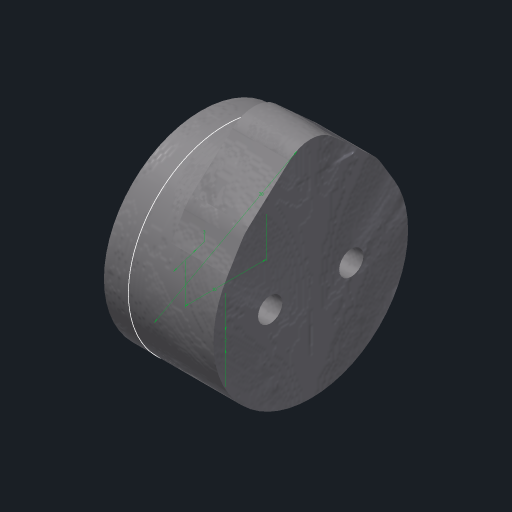
# Autodesk Inventor part: CIRCULAR_FIN_DE_CARRERA
Saved by Autodesk Inventor 2024.3 (Build 283343000, 343)
## iProperties
Created: 2024-07-21
Part Number: CIRCULAR_FIN_DE_CARRERA
Material: Steel, Mild, Welded
Document SubType Name: Modeling
Designer: Niler
Density: 7.85 g/cm^3
Appearance: Weld - Steel Mild
Author: Niler
Autodesk Inventor part; units mm, degrees
ref_plane "YZ Plane" through (0, 0, 0) normal (1, 0, 0) x (0, 1, 0)
ref_plane "XZ Plane" through (0, 0, 0) normal (0, 1, 0) x (-1, 0, 0)
ref_plane "XY Plane" through (0, 0, 0) normal (0, 0, 1) x (1, 0, 0)
sketch "Sketch1" plane through (0, 0, 0) normal (1, 0, 0) x (0, 1, 0)
  circle A0 centre (0, 0) radius 10
  circle A1 centre (0, 0) radius 12
  circle A2 centre (0, 5) radius 1.5
  circle A3 centre (0, -5) radius 1.5
  line L0 (0, 5) -> (0, -5) construction
  dimension "d0" = 20
  dimension "d1" = 2
  dimension "d2" = 3
  dimension "d3" = 10
  constraints: 4 centre point, 2 coincident, 2 end point, 1 equal radius, 1 midpoint, 1 vertical, 1 vertical alignment
  measures "d0" diameter of A0
  measures "d1" radial gap between concentric circles of A0 A1
  measures "d2" diameter of A2
  measures "d3" distance of L0.start L0.end
extrude "Extrusion1" add sketch "Sketch1" along normal blind 3.5 contours A0 | A1
extrude "Extrusion2" add sketch "Sketch1" against normal blind 3 contours A1
sketch "Sketch2" plane through (3.5, 0, 0) normal (1, 0, 0) x (0, 0, -1)
  circle A0 centre (0, 0) radius 12 projected
  circle A1 centre (-5, 0) radius 1.5 projected
  circle A2 centre (5, 0) radius 1.5 projected
  circle A3 centre (0, 11.8) radius 3.9
  circle A4 centre (0, 0) radius 12 projected
  line L0 (-10.2593, 6.2247) -> (-8.5634, 9.0198)
  line L1 (-7.6474, 10.1301) -> (-2.6198, 14.6891)
  arc A5 (-7.6474, 10.1301) -> (-8.5634, 9.0198) centre (-4.2887, 6.4262) ccw
  line L2 (0, 0) -> (0, 4.7438)
  line L3 (10.2593, 6.2247) -> (8.5634, 9.0198)
  line L4 (7.6474, 10.1301) -> (2.6198, 14.6891)
  arc A6 (8.5634, 9.0198) -> (7.6474, 10.1301) centre (4.2887, 6.4262) ccw
  point P0 (0.4335, 15.6758)
  point P1 (10.2649, 6.2155)
  point P2 (-10.2593, 6.2247)
  point P3 (10.2593, 6.2247)
  point P4 (-3.8748, 11.3572)
  point P5 (3.8748, 11.3572)
  dimension "d10" = 5
  dimension "d11" = 11.8
  dimension "d12" = 7.8
  constraints: 10 end point, 7 point on circle, 5 symmetric about line, 4 tangent, 3 centre point, 1 vertical, 1 vertical alignment, 3 other
  measures "d10" radius of A5
  measures "d11" distance of point (0, 0) A3.centre
  measures "d12" diameter of A3
extrude "Extrusion3" add sketch "Sketch2" along normal blind 7
body "Solid1"
